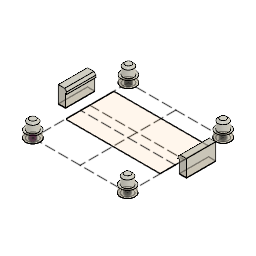
0.96_OLED_template_v4 (Autodesk Fusion 360 design; units mm, degrees)
Autodesk Fusion 360 part; units mm, degrees
note: some values were not read from the file. Chosen so that the rebuilt part matches the saved one: which bodies a step acts on.
sketch "Sketch1" plane through (0, 0, 0) normal (0, 0, 1) x (1, 0, 0)
  line L0 (0, 0) -> (22.6, 0) construction
  line L1 (22.6, 0) -> (22.6, 22.8) construction
  line L2 (22.6, 22.8) -> (0, 22.8) construction
  line L3 (0, 22.8) -> (0, 0) construction
  circle A0 centre (0, 22.8) radius 1.75
  circle A1 centre (0, 22.8) radius 1.25
  line L4 (11.3, 22.8) -> (11.3, 0) construction
  line L5 (22.6, 11.4) -> (0, 11.4) construction
  circle A2 centre (22.6, 22.8) radius 1.75
  circle A3 centre (22.6, 22.8) radius 1.25
  circle A4 centre (0, 0) radius 1.25
  circle A5 centre (0, 0) radius 1.75
  circle A6 centre (22.6, 0) radius 1.75
  circle A7 centre (22.6, 0) radius 1.25
  line L6 (0.05, 19.3) -> (22.55, 19.3)
  line L7 (22.55, 19.3) -> (22.55, 7.8)
  line L8 (22.55, 7.8) -> (0.05, 7.8)
  line L9 (0.05, 7.8) -> (0.05, 19.3)
  line L10 (0.05, 13.55) -> (22.55, 13.55) construction
  line L11 (-4, 17.05) -> (-2.25, 17.05)
  line L12 (-2.25, 17.05) -> (-2.25, 10.05)
  line L13 (-2.25, 10.05) -> (-4, 10.05)
  line L14 (-4, 10.05) -> (-4, 17.05)
  line L15 (24.85, 17.05) -> (24.85, 10.05)
  line L16 (26.6, 17.05) -> (24.85, 17.05)
  line L17 (26.6, 10.05) -> (26.6, 17.05)
  line L18 (24.85, 10.05) -> (26.6, 10.05)
  dimension "d1" = 22.8
  dimension "d2" = 22.6
  dimension "d3" = 3.5
  dimension "d4" = 2.5
  dimension "d5" = 22.5
  dimension "d6" = 11.5
  dimension "d7" = 3.5
  dimension "d8" = 1.75
  dimension "d9" = 7
  dimension "d10" = 2.25
  measures "d3" diameter of A0
  measures "d4" diameter of A1
  measures "d7" distance of L2 L6
  measures "d10" distance of L3 L12
extrude "Extrude1" add sketch "Sketch1" along normal blind 4 contours A1 | A3 | A4 | A7 makes body 1 at (1.2484, -0.0623, 2.6667) makes body 2 at (1.2484, 22.7377, 2.6667) makes body 3 at (23.8484, 22.7377, 2.6667) makes body 4 at (23.8484, -0.0623, 2.6667)
extrude "Extrude2" add sketch "Sketch1" along normal blind 1.7 contours A0 | A2 | A5 | A6 bodies 3 1 2 4
chamfer "Chamfer1" distance 0.5 angle 45 4 edges at (-1.1654, -0.452, 4) (-1.1654, 22.348, 4) (21.4346, -0.452, 4) (21.4346, 22.348, 4) on bodies 1 2 3 4
extrude "Extrude3" add sketch "Sketch1" along normal blind 4 separate body contours L11 L12 L13 L14 | L15 L16 L17 L18 makes body 5 at (-2.25, 14.7167, 2.6667) makes body 6 at (26.6, 12.3833, 1.3333)
sketch "Sketch2" plane through (-2.25, 0, 0) normal (1, 0, 0) x (0, 1, 0)
  line L0 (10.05, 0) -> (17.05, 0)
  line L1 (17.05, 0) -> (17.05, 4)
  line L2 (17.05, 4) -> (10.05, 4)
  line L3 (10.05, 4) -> (10.05, 0)
  line L4 (10.05, 4) -> (17.05, 4)
  line L5 (17.05, 4) -> (17.05, 3)
  line L6 (17.05, 3) -> (10.05, 3)
  line L7 (10.05, 3) -> (10.05, 4)
  dimension "d18" = 1
extrude "Extrude4" add sketch "Sketch2" along normal blind 0.3 contours L1 L2 L3 L4 L5 L6 L7 bodies 5
sketch "Sketch3" plane through (24.85, 0, 0) normal (-1, 0, 0) x (0, -1, 0)
  line L0 (-17.05, 0) -> (-10.05, 0)
  line L1 (-10.05, 0) -> (-10.05, 4)
  line L2 (-10.05, 4) -> (-17.05, 4)
  line L3 (-17.05, 4) -> (-17.05, 0)
  line L4 (-17.05, 4) -> (-10.05, 4)
  line L5 (-10.05, 4) -> (-10.05, 3)
  line L6 (-10.05, 3) -> (-17.05, 3)
  line L7 (-17.05, 3) -> (-17.05, 4)
  dimension "d21" = 1
extrude "Extrude5" add sketch "Sketch3" along normal blind 0.3 contours L1 L2 L3 L4 L5 L6 L7 bodies 6
chamfer "Chamfer2" distance 0.5 angle 45 1 edges at (24.55, 13.55, 4) on bodies 6
chamfer "Chamfer3" distance 0.5 angle 45 1 edges at (-1.95, 13.55, 4) on bodies 5
